Autodesk Inventor part; units mm, degrees
(part 2 of 2)
extrude "Extrusion14" add sketch "Sketch20" along normal blind 2.54 contours L123 L124 L125 L126 L127 L128 L129 L130 L131 L132 L133 L134 | L151 L152 L153 L154 L155 L156 | L181 L182 L183 L184 L185 L186 | L204 L197 L198 L199 L200 L201 L202 L203 | S194 S179 A0 | A0 S179 S180 S181 S182 S183 S184 L205 L206 S185 S186 S187 S188 S189 S190 S191 S192 L207 L208 S193 S194 | S73 S74 S75 S76 S77 S78 L135 L136 S79 S80 S81 S82 S83 S84 S85 S86 L137 L138 S87 S88 A0 | A0 S88 S73 | S92 S93 S94 S95 S96 S89 S90 S91 A0 | A0 S91 S92 | S167 S168 A0 | A0 S168 S169 S170 S171 S172 S165 S166 S167 | S153 S154 A0 | A0 S154 S155 S156 S157 S158 S151 S152 S153 | S103 L157 L158 S104 S105 S106 S107 S108 S109 S110 S111 L159 L160 S112 S113 S114 S115 S116 S117 S118 A0 | A0 S118 S103 | S150 S135 A0 | A0 S135 S136 S137 S138 S139 S140 L165 L166 S141 S142 S143 S144 S145 S146 S147 S148 L167 L168 S149 S150 | S119 L161 L162 S120 S121 S122 S123 S124 S125 S126 S127 L163 L164 S128 S129 S130 S131 S132 S133 S134 A0 | A0 S134 S119 | S0 S1 L0 L1 L2 L3 L4 S2 S3 | L8 L9 L10 L11 L12 L13 L14 L15 L16 L17 L18 L19 | L20 L21 L22 L23 L24 L25 L26 L27 L28 L29 L30 L31 | L32 L33 L34 L35 L36 L37 L38 S8 S9 S10 L39 | L43 L44 L45 L46 L47 L48 L49 L50 | L54 L55 L56 L57 L58 L59 L60 L61 L62 L63 L64 L65 L66 | L67 L68 L69 L70 L71 L72 L73 L74 | L78 L79 L80 L81 L82 L83 L84 S15 S16 S17 L85 | S22 S23 L89 L90 L91 S24 S25 | L95 L96 S30 S31 S32 S33 S34 S35 L97 L98 S36 S37 S38 S39 S40 L99 L100 | S41 S42 S43 S44 | L101 L102 L103 L104 L105 L106 S53 L107 L108 L109 L110 | S54 S55 S56 L111 S57 S58 S59 S60 L112 S61 S62 | L113 L114 L115 L116 L117 L118 L119 L120 L121 L122 | L139 L140 L141 L142 L143 L144 L145 L146 L147 L148 L149 L150 | L169 L170 L171 L172 L173 L174 L175 L176 L177 L178 L179 L180 | L187 L188 L189 L190 L191 L192 L193 L194 L195 L196
fillet "Fillet1" radius 1.5875 22 edges at (29.21, 35.6826, 12.8193) (29.21, 39.0904, 11.1154) (29.21, 35.1147, 3.164) (29.21, 27.0816, 4.7099) (29.21, 27.0816, 9.4724) (29.21, 35.0208, -3.0926) (29.21, 36.3276, -12.676) (29.21, 39.5946, -10.7157) (29.21, 26.9748, -9.6449) (29.21, 26.9748, -4.89) (29.21, 22.7602, -4.568) (29.21, 19.5798, 4.9096) (29.21, -12.3825, 4.699) (29.21, -12.3825, 9.271) (29.21, -12.3237, -9.2739) (29.21, -20.5787, -9.2739) (29.21, -20.6375, 4.699) (29.21, -20.5787, -4.7019) (29.21, -20.6375, 9.271) (29.21, -12.3237, -4.7019) (29.21, -25.4, -4.7625) (29.21, -25.4, 4.7625)
fillet "Fillet2" radius 3.175 1 edges at (25.4, -104.7779, 0)
fillet "Fillet3" radius 3.175 1 edges at (0, -104.7779, 0)
fillet "Fillet4" radius 1.5875 1 edges at (29.21, 43.18, 14.4399)
fillet "Fillet5" radius 1.5875 1 edges at (29.21, 43.18, -16.0401)
fillet "Fillet6" radius 1.5875 1 edges at (29.21, 7.62, 14.4272)
fillet "Fillet7" radius 1.5875 1 edges at (29.21, 7.62, -16.0528)
fillet "Fillet8" radius 1.5875 1 edges at (29.21, -40.005, 14.4272)
fillet "Fillet9" radius 1.5875 1 edges at (29.21, -40.005, -16.0528)
fillet "Fillet10" radius 1.5875 1 edges at (29.21, -4.445, -16.0528)
fillet "Fillet11" radius 1.5875 1 edges at (29.21, -4.445, 14.4272)
body "Solid1"
